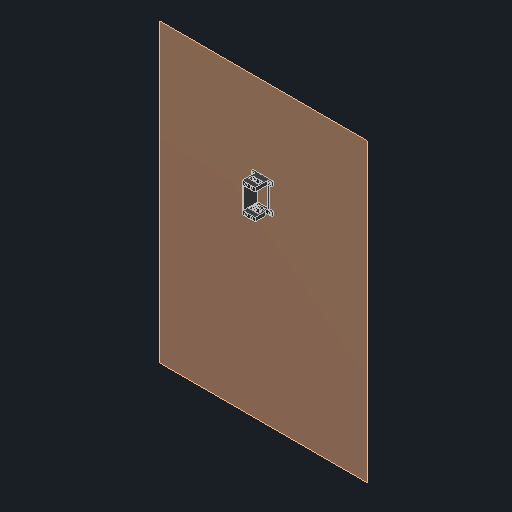
# Autodesk Inventor part: yaw_motor_mount
Saved by Autodesk Inventor 2026.1 (Build 301233020, 233B)
## iProperties
Created: 2025-11-24
Part Number: yaw_motor_mount
Material: 고무, 검은색
Document SubType Name: Modeling
Designer: jaewook
Density: 0.93 g/cm^3
Appearance: 고무 - 검은색
Author: jaewook
Autodesk Inventor part; units mm, degrees
ref_plane "YZ Plane" through (0, 0, 0) normal (1, 0, 0) x (0, 1, 0)
ref_plane "XZ Plane" through (0, 0, 0) normal (0, 1, 0) x (-1, 0, 0)
ref_plane "XY Plane" through (0, 0, 0) normal (0, 0, 1) x (1, 0, 0)
ref_plane "작업 평면1" through (0, 0, -71.9624) normal (0, 0, 1) x (1, 0, 0)
sketch "스케치1" plane through (0, 0, -71.9624) normal (0, 0, 1) x (1, 0, 0)
  line L0 (10, 115.2) -> (10, 75.2) construction
  line L1 (-10, 75.2) -> (-10, 115.2) construction
  line L2 (-10, 115.2) -> (10, 115.2) construction
  line L3 (10, 122.7) -> (-10, 122.7) construction
  line L4 (10, 115.2) -> (10, 122.7) construction
  line L5 (-10, 122.7) -> (-10, 115.2) construction
  circle A0 centre (-4.9, 119.5) radius 2.5 construction
  circle A1 centre (5, 119.5) radius 2.5 construction
  circle A2 centre (5, 70.9) radius 2.5 construction
  circle A3 centre (-4.9, 70.9) radius 2.5 construction
  line L6 (10, 75.2) -> (10, 67.7) construction
  line L7 (10, 67.7) -> (-10, 67.7) construction
  line L8 (-10, 67.7) -> (-10, 75.2) construction
  line L9 (10, 115.2) -> (10, 75.2) projected
  line L10 (-10, 75.2) -> (-10, 115.2) projected
  line L11 (-10, 122.7) -> (-10, 115.2) projected
  line L12 (-10, 115.2) -> (10, 115.2) projected
  line L13 (10, 115.2) -> (10, 122.7) projected
  line L14 (10, 122.7) -> (-10, 122.7) projected
  line L15 (-10, 67.7) -> (-10, 75.2) projected
  line L16 (10, 67.7) -> (-10, 67.7) projected
  line L17 (10, 75.2) -> (10, 67.7) projected
  circle A4 centre (-4.9, 70.9) radius 2.5 projected
  circle A5 centre (5, 70.9) radius 2.5 projected
  line L18 (10, 75.2) -> (-10, 75.2) projected
  circle A6 centre (5, 119.5) radius 2.5 projected
  circle A7 centre (-4.9, 119.5) radius 2.5 projected
  point P0 (0, 0)
ref_plane "작업 평면2" through (0, 0, -71.9624) normal (0, 0, 1) x (1, 0, 0)
sketch "스케치2" plane through (0, 0, -71.9624) normal (0, 0, 1) x (1, 0, 0)
  circle A0 centre (0, 170) radius 2 projected
  circle A1 centre (-73.6122, 42.5) radius 2 projected
  circle A2 centre (73.6122, 42.5) radius 2 projected
  line L0 (-175, 220) -> (-175, 200) projected
  line L1 (-175, 200) -> (-130, 200) projected
  line L2 (-130, 200) -> (-130, 105) projected
  line L3 (-130, 105) -> (-175, 105) projected
  line L4 (-175, 105) -> (-175, -105) projected
  line L5 (-175, -105) -> (-130, -105) projected
  line L6 (-130, -105) -> (-130, -200) projected
  line L7 (-130, -200) -> (-175, -200) projected
  line L8 (-175, -200) -> (-175, -220) projected
  arc A3 (-175, -220) -> (-145, -250) centre (-145, -220) ccw projected
  line L9 (-145, -250) -> (145, -250) projected
  arc A4 (145, -250) -> (175, -220) centre (145, -220) ccw projected
  line L10 (175, -220) -> (175, -200) projected
  line L11 (175, -200) -> (130, -200) projected
  line L12 (130, -200) -> (130, -105) projected
  line L13 (130, -105) -> (175, -105) projected
  line L14 (175, -105) -> (175, 105) projected
  line L15 (175, 105) -> (130, 105) projected
  line L16 (130, 105) -> (130, 200) projected
  line L17 (130, 200) -> (175, 200) projected
  line L18 (175, 200) -> (175, 220) projected
  arc A5 (175, 220) -> (145, 250) centre (145, 220) ccw projected
  line L19 (145, 250) -> (-145, 250) projected
  arc A6 (-145, 250) -> (-175, 220) centre (-145, 220) ccw projected
  circle A7 centre (0, 170) radius 2 projected
  circle A8 centre (-73.6122, 42.5) radius 2 projected
  circle A9 centre (73.6122, 42.5) radius 2 projected
  line L20 (-175, 220) -> (-175, 200) projected
  line L21 (-175, 200) -> (-130, 200) projected
  line L22 (-130, 200) -> (-130, 105) projected
  line L23 (-130, 105) -> (-175, 105) projected
  line L24 (-175, 105) -> (-175, -105) projected
  line L25 (-175, -105) -> (-130, -105) projected
  line L26 (-130, -105) -> (-130, -200) projected
  line L27 (-130, -200) -> (-175, -200) projected
  line L28 (-175, -200) -> (-175, -220) projected
  arc A10 (-175, -220) -> (-145, -250) centre (-145, -220) ccw projected
  line L29 (-145, -250) -> (145, -250) projected
  arc A11 (145, -250) -> (175, -220) centre (145, -220) ccw projected
  line L30 (175, -220) -> (175, -200) projected
  line L31 (175, -200) -> (130, -200) projected
  line L32 (130, -200) -> (130, -105) projected
  line L33 (130, -105) -> (175, -105) projected
  line L34 (175, -105) -> (175, 105) projected
  line L35 (175, 105) -> (130, 105) projected
  line L36 (130, 105) -> (130, 200) projected
  line L37 (130, 200) -> (175, 200) projected
  line L38 (175, 200) -> (175, 220) projected
  arc A12 (175, 220) -> (145, 250) centre (145, 220) ccw projected
  line L39 (145, 250) -> (-145, 250) projected
  arc A13 (-145, 250) -> (-175, 220) centre (-145, 220) ccw projected
  circle A14 centre (0, 170) radius 2 projected
  circle A15 centre (-73.6122, 42.5) radius 2 projected
  circle A16 centre (73.6122, 42.5) radius 2 projected
  line L40 (-175, 220) -> (-175, 200) projected
  line L41 (-175, 200) -> (-130, 200) projected
  line L42 (-130, 200) -> (-130, 105) projected
  line L43 (-130, 105) -> (-175, 105) projected
  line L44 (-175, 105) -> (-175, -105) projected
  line L45 (-175, -105) -> (-130, -105) projected
  line L46 (-130, -105) -> (-130, -200) projected
  line L47 (-130, -200) -> (-175, -200) projected
  line L48 (-175, -200) -> (-175, -220) projected
  arc A17 (-175, -220) -> (-145, -250) centre (-145, -220) ccw projected
  line L49 (-145, -250) -> (145, -250) projected
  arc A18 (145, -250) -> (175, -220) centre (145, -220) ccw projected
  line L50 (175, -220) -> (175, -200) projected
  line L51 (175, -200) -> (130, -200) projected
  line L52 (130, -200) -> (130, -105) projected
  line L53 (130, -105) -> (175, -105) projected
  line L54 (175, -105) -> (175, 105) projected
  line L55 (175, 105) -> (130, 105) projected
  line L56 (130, 105) -> (130, 200) projected
  line L57 (130, 200) -> (175, 200) projected
  line L58 (175, 200) -> (175, 220) projected
  arc A19 (175, 220) -> (145, 250) centre (145, 220) ccw projected
  line L59 (145, 250) -> (-145, 250) projected
  arc A20 (-145, 250) -> (-175, 220) centre (-145, 220) ccw projected
  circle A21 centre (-4.9, 70.9) radius 2.5 projected
  circle A22 centre (-4.9, 70.9) radius 2.5 projected
  circle A23 centre (5, 70.9) radius 2.5 projected
  circle A24 centre (5, 119.5) radius 2.5 projected
  circle A25 centre (-4.9, 119.5) radius 2.5 projected
  arc A26 (175, 220) -> (145, 250) centre (145, 220) ccw projected
  line L60 (-145, 250) -> (145, 250) projected
  arc A27 (-145, 250) -> (-175, 220) centre (-145, 220) ccw projected
  line L61 (-175, -220) -> (-175, 220) projected
  arc A28 (-175, -220) -> (-145, -250) centre (-145, -220) ccw projected
  line L62 (145, -250) -> (-145, -250) projected
  arc A29 (145, -250) -> (175, -220) centre (145, -220) ccw projected
  line L63 (175, 220) -> (175, -220) projected
  circle A30 centre (0, -175) radius 36 projected
  circle A31 centre (0, 85) radius 103.75 projected
  line L64 (10, 75.2) -> (-10, 75.2)
  line L65 (-10, 75.2) -> (-10, 115.2)
  line L66 (-10, 115.2) -> (10, 115.2)
  line L67 (10, 115.2) -> (10, 75.2)
  line L68 (10.3, 74.9) -> (10.3, 115.5)
  line L69 (10.3, 115.5) -> (-10.3, 115.5)
  line L70 (-10.3, 115.5) -> (-10.3, 74.9)
  line L71 (-10.3, 74.9) -> (10.3, 74.9)
  line L72 (12, 67.7) -> (-12, 67.7)
  line L73 (-12, 67.7) -> (-12, 122.7)
  line L74 (-12, 122.7) -> (12, 122.7)
  line L75 (12, 122.7) -> (12, 67.7)
  line L76 (10, 95.2) -> (-10, 95.2) construction
  line L77 (0, 95.2) -> (0, 75.2) construction
  line L78 (10.3, 74.9) -> (12, 74.9)
  line L79 (10.3, 115.5) -> (12, 115.5)
  circle A32 centre (-4.9, 119.5) radius 2
  circle A33 centre (5, 119.5) radius 2
  circle A34 centre (-4.9, 70.9) radius 2
  circle A35 centre (5, 70.9) radius 2
  circle A36 centre (-123, 166.7672) radius 2 projected
  circle A37 centre (122.9975, 135.7594) radius 2 projected
  circle A38 centre (97.9975, -135.761) radius 2 projected
  circle A39 centre (15.5, 71.3) radius 2 projected
  circle A40 centre (165.0067, -210) radius 2.5 projected
  circle A41 centre (119.0003, -180.2596) radius 1.25 projected
  circle A42 centre (-119, -122.2672) radius 1.25 projected
  circle A43 centre (-123, -135.7672) radius 2 projected
  circle A44 centre (0.0196, 140) radius 2 projected
  circle A45 centre (-123, -166.7672) radius 2 projected
  circle A46 centre (-70, -122.2672) radius 1.25 projected
  circle A47 centre (69.9966, -122.2627) radius 1.25 projected
  circle A48 centre (-165, 0) radius 2.5 projected
  circle A49 centre (-165.0067, 210) radius 2.5 projected
  circle A50 centre (-15.5, 119.1) radius 2 projected
  circle A51 centre (97.9995, -166.761) radius 2 projected
  circle A52 centre (97.9995, 166.761) radius 2 projected
  circle A53 centre (-98, 166.7672) radius 2 projected
  circle A54 centre (-123, 135.7672) radius 2 projected
  circle A55 centre (97.9975, 135.761) radius 2 projected
  circle A56 centre (122.9975, -135.7594) radius 2 projected
  circle A57 centre (-15.5, 71.3) radius 2 projected
  circle A58 centre (-164.9933, -210) radius 2.5 projected
  circle A59 centre (70.0003, -180.2627) radius 1.25 projected
  circle A60 centre (-119, -180.2672) radius 1.25 projected
  circle A61 centre (-98, -135.7672) radius 2 projected
  circle A62 centre (47.6216, 57.483) radius 2 projected
  circle A63 centre (-47.6412, 57.517) radius 2 projected
  circle A64 centre (-98, -166.7672) radius 2 projected
  circle A65 centre (-70, -180.2672) radius 1.25 projected
  circle A66 centre (118.9966, -122.2596) radius 1.25 projected
  circle A67 centre (165, 0) radius 2.5 projected
  circle A68 centre (164.9933, 210) radius 2.5 projected
  circle A69 centre (15.5, 119.1) radius 2 projected
  circle A70 centre (122.9995, -166.7594) radius 2 projected
  circle A71 centre (122.9995, 166.7594) radius 2 projected
  circle A72 centre (-98, 135.7672) radius 2 projected
  circle A73 centre (-123, 166.7672) radius 2 projected
  circle A74 centre (122.9975, 135.7594) radius 2 projected
  circle A75 centre (97.9975, -135.761) radius 2 projected
  circle A76 centre (15.5, 71.3) radius 2 projected
  circle A77 centre (165.0067, -210) radius 2.5 projected
  circle A78 centre (119.0003, -180.2596) radius 1.25 projected
  circle A79 centre (-119, -122.2672) radius 1.25 projected
  circle A80 centre (-123, -135.7672) radius 2 projected
  circle A81 centre (0.0196, 140) radius 2 projected
  circle A82 centre (-123, -166.7672) radius 2 projected
  circle A83 centre (-70, -122.2672) radius 1.25 projected
  circle A84 centre (69.9966, -122.2627) radius 1.25 projected
  circle A85 centre (-165, 0) radius 2.5 projected
  circle A86 centre (-165.0067, 210) radius 2.5 projected
  circle A87 centre (-15.5, 119.1) radius 2 projected
  circle A88 centre (97.9995, -166.761) radius 2 projected
  circle A89 centre (97.9995, 166.761) radius 2 projected
  circle A90 centre (-98, 166.7672) radius 2 projected
  circle A91 centre (-123, 135.7672) radius 2 projected
  circle A92 centre (97.9975, 135.761) radius 2 projected
  circle A93 centre (122.9975, -135.7594) radius 2 projected
  circle A94 centre (-15.5, 71.3) radius 2 projected
  circle A95 centre (-164.9933, -210) radius 2.5 projected
  circle A96 centre (70.0003, -180.2627) radius 1.25 projected
  circle A97 centre (-119, -180.2672) radius 1.25 projected
  circle A98 centre (-98, -135.7672) radius 2 projected
  circle A99 centre (47.6216, 57.483) radius 2 projected
  circle A100 centre (-47.6412, 57.517) radius 2 projected
  circle A101 centre (-98, -166.7672) radius 2 projected
  circle A102 centre (-70, -180.2672) radius 1.25 projected
  circle A103 centre (118.9966, -122.2596) radius 1.25 projected
  circle A104 centre (165, 0) radius 2.5 projected
  circle A105 centre (164.9933, 210) radius 2.5 projected
  circle A106 centre (15.5, 119.1) radius 2 projected
  circle A107 centre (122.9995, -166.7594) radius 2 projected
  circle A108 centre (122.9995, 166.7594) radius 2 projected
  circle A109 centre (-98, 135.7672) radius 2 projected
  circle A110 centre (-123, 166.7672) radius 2 projected
  circle A111 centre (122.9975, 135.7594) radius 2 projected
  circle A112 centre (97.9975, -135.761) radius 2 projected
  circle A113 centre (15.5, 71.3) radius 2 projected
  circle A114 centre (165.0067, -210) radius 2.5 projected
  circle A115 centre (119.0003, -180.2596) radius 1.25 projected
  circle A116 centre (-119, -122.2672) radius 1.25 projected
  circle A117 centre (-123, -135.7672) radius 2 projected
  circle A118 centre (0.0196, 140) radius 2 projected
  circle A119 centre (-123, -166.7672) radius 2 projected
  circle A120 centre (-70, -122.2672) radius 1.25 projected
  circle A121 centre (69.9966, -122.2627) radius 1.25 projected
  circle A122 centre (-165, 0) radius 2.5 projected
  circle A123 centre (-165.0067, 210) radius 2.5 projected
  circle A124 centre (-15.5, 119.1) radius 2 projected
  circle A125 centre (97.9995, -166.761) radius 2 projected
  circle A126 centre (97.9995, 166.761) radius 2 projected
  circle A127 centre (-98, 166.7672) radius 2 projected
  circle A128 centre (-123, 135.7672) radius 2 projected
  circle A129 centre (97.9975, 135.761) radius 2 projected
  circle A130 centre (122.9975, -135.7594) radius 2 projected
  circle A131 centre (-15.5, 71.3) radius 2 projected
  circle A132 centre (-164.9933, -210) radius 2.5 projected
  circle A133 centre (70.0003, -180.2627) radius 1.25 projected
  circle A134 centre (-119, -180.2672) radius 1.25 projected
  circle A135 centre (-98, -135.7672) radius 2 projected
  circle A136 centre (47.6216, 57.483) radius 2 projected
  circle A137 centre (-47.6412, 57.517) radius 2 projected
  circle A138 centre (-98, -166.7672) radius 2 projected
  circle A139 centre (-70, -180.2672) radius 1.25 projected
  circle A140 centre (118.9966, -122.2596) radius 1.25 projected
  circle A141 centre (165, 0) radius 2.5 projected
  circle A142 centre (164.9933, 210) radius 2.5 projected
  circle A143 centre (15.5, 119.1) radius 2 projected
  circle A144 centre (122.9995, -166.7594) radius 2 projected
  circle A145 centre (122.9995, 166.7594) radius 2 projected
  circle A146 centre (-98, 135.7672) radius 2 projected
  line L80 (-110, 97.5) -> (-93, 97.5) projected
  line L81 (-93, 97.5) -> (-93, 89.5) projected
  line L82 (-93, 89.5) -> (-110, 89.5) projected
  line L83 (-110, 89.5) -> (-110, 97.5) projected
  circle A147 centre (148, -23.75) radius 2 projected
  circle A148 centre (130.626, -27.584) radius 1.5 projected
  circle A149 centre (118.5, 61.5) radius 1.5 projected
  circle A150 centre (-118.5, 61.5) radius 1.5 projected
  circle A151 centre (21, -158.9548) radius 2 projected
  circle A152 centre (-22, -53) radius 2 projected
  circle A153 centre (-49.5, -194.9548) radius 2 projected
  circle A154 centre (-49.5, -158.9548) radius 2 projected
  circle A155 centre (21, -194.9548) radius 2 projected
  circle A156 centre (-155, 25) radius 1.5 projected
  circle A157 centre (118.5, 25) radius 1.5 projected
  circle A158 centre (123.133, -76) radius 1.5 projected
  circle A159 centre (37, -84) radius 2 projected
  line L84 (-93, -89.5) -> (-93, -97.5) projected
  line L85 (-93, -97.5) -> (-110, -97.5) projected
  line L86 (-110, -97.5) -> (-110, -89.5) projected
  line L87 (-110, -89.5) -> (-93, -89.5) projected
  circle A160 centre (-130, 5) radius 6 projected
  line L88 (110, 89.5) -> (93, 89.5) projected
  line L89 (93, 89.5) -> (93, 97.5) projected
  line L90 (93, 97.5) -> (110, 97.5) projected
  line L91 (110, 97.5) -> (110, 89.5) projected
  circle A161 centre (148, -84) radius 2 projected
  circle A162 centre (47.999, -27.584) radius 1.5 projected
  circle A163 centre (155, 61.5) radius 1.5 projected
  circle A164 centre (-155, 61.5) radius 1.5 projected
  circle A165 centre (49.5, -158.9548) radius 2 projected
  circle A166 centre (-86, -93.5) radius 2 projected
  circle A167 centre (-21, -194.9548) radius 2 projected
  circle A168 centre (-150, -53) radius 2 projected
  circle A169 centre (-21, -158.9548) radius 2 projected
  circle A170 centre (49.5, -194.9548) radius 2 projected
  circle A171 centre (-118.5, 25) radius 1.5 projected
  circle A172 centre (155, 25) radius 1.5 projected
  circle A173 centre (48, -76) radius 1.5 projected
  circle A174 centre (37, -23.75) radius 2 projected
  line L92 (110, -89.5) -> (110, -97.5) projected
  line L93 (110, -97.5) -> (93, -97.5) projected
  line L94 (93, -97.5) -> (93, -89.5) projected
  line L95 (93, -89.5) -> (110, -89.5) projected
  circle A175 centre (-70, 5) radius 6 projected
  line L96 (-110, 97.5) -> (-93, 97.5) projected
  line L97 (-93, 97.5) -> (-93, 89.5) projected
  line L98 (-93, 89.5) -> (-110, 89.5) projected
  line L99 (-110, 89.5) -> (-110, 97.5) projected
  circle A176 centre (148, -23.75) radius 2 projected
  circle A177 centre (130.626, -27.584) radius 1.5 projected
  circle A178 centre (118.5, 61.5) radius 1.5 projected
  circle A179 centre (-118.5, 61.5) radius 1.5 projected
  circle A180 centre (21, -158.9548) radius 2 projected
  circle A181 centre (-22, -53) radius 2 projected
  circle A182 centre (-49.5, -194.9548) radius 2 projected
  circle A183 centre (-49.5, -158.9548) radius 2 projected
  circle A184 centre (21, -194.9548) radius 2 projected
  circle A185 centre (-155, 25) radius 1.5 projected
  circle A186 centre (118.5, 25) radius 1.5 projected
  circle A187 centre (123.133, -76) radius 1.5 projected
  circle A188 centre (37, -84) radius 2 projected
  line L100 (-93, -89.5) -> (-93, -97.5) projected
  line L101 (-93, -97.5) -> (-110, -97.5) projected
  line L102 (-110, -97.5) -> (-110, -89.5) projected
  line L103 (-110, -89.5) -> (-93, -89.5) projected
  circle A189 centre (-130, 5) radius 6 projected
  line L104 (110, 89.5) -> (93, 89.5) projected
  line L105 (93, 89.5) -> (93, 97.5) projected
  line L106 (93, 97.5) -> (110, 97.5) projected
  line L107 (110, 97.5) -> (110, 89.5) projected
  circle A190 centre (148, -84) radius 2 projected
  circle A191 centre (47.999, -27.584) radius 1.5 projected
  circle A192 centre (155, 61.5) radius 1.5 projected
  circle A193 centre (-155, 61.5) radius 1.5 projected
  circle A194 centre (49.5, -158.9548) radius 2 projected
  circle A195 centre (-86, -93.5) radius 2 projected
  circle A196 centre (-21, -194.9548) radius 2 projected
  circle A197 centre (-150, -53) radius 2 projected
  circle A198 centre (-21, -158.9548) radius 2 projected
  circle A199 centre (49.5, -194.9548) radius 2 projected
  circle A200 centre (-118.5, 25) radius 1.5 projected
  circle A201 centre (155, 25) radius 1.5 projected
  circle A202 centre (48, -76) radius 1.5 projected
  circle A203 centre (37, -23.75) radius 2 projected
  line L108 (110, -89.5) -> (110, -97.5) projected
  line L109 (110, -97.5) -> (93, -97.5) projected
  line L110 (93, -97.5) -> (93, -89.5) projected
  line L111 (93, -89.5) -> (110, -89.5) projected
  circle A204 centre (-70, 5) radius 6 projected
  line L112 (-110, 97.5) -> (-93, 97.5) projected
  line L113 (-93, 97.5) -> (-93, 89.5) projected
  line L114 (-93, 89.5) -> (-110, 89.5) projected
  line L115 (-110, 89.5) -> (-110, 97.5) projected
  circle A205 centre (148, -23.75) radius 2 projected
  circle A206 centre (130.626, -27.584) radius 1.5 projected
  circle A207 centre (118.5, 61.5) radius 1.5 projected
  circle A208 centre (-118.5, 61.5) radius 1.5 projected
  circle A209 centre (21, -158.9548) radius 2 projected
  circle A210 centre (-22, -53) radius 2 projected
  circle A211 centre (-49.5, -194.9548) radius 2 projected
  circle A212 centre (-49.5, -158.9548) radius 2 projected
  circle A213 centre (21, -194.9548) radius 2 projected
  circle A214 centre (-155, 25) radius 1.5 projected
  circle A215 centre (118.5, 25) radius 1.5 projected
  circle A216 centre (123.133, -76) radius 1.5 projected
  circle A217 centre (37, -84) radius 2 projected
  line L116 (-93, -89.5) -> (-93, -97.5) projected
  line L117 (-93, -97.5) -> (-110, -97.5) projected
  line L118 (-110, -97.5) -> (-110, -89.5) projected
  line L119 (-110, -89.5) -> (-93, -89.5) projected
  circle A218 centre (-130, 5) radius 6 projected
  line L120 (110, 89.5) -> (93, 89.5) projected
  line L121 (93, 89.5) -> (93, 97.5) projected
  line L122 (93, 97.5) -> (110, 97.5) projected
  line L123 (110, 97.5) -> (110, 89.5) projected
  circle A219 centre (148, -84) radius 2 projected
  circle A220 centre (47.999, -27.584) radius 1.5 projected
  circle A221 centre (155, 61.5) radius 1.5 projected
  circle A222 centre (-155, 61.5) radius 1.5 projected
  circle A223 centre (49.5, -158.9548) radius 2 projected
  circle A224 centre (-86, -93.5) radius 2 projected
  circle A225 centre (-21, -194.9548) radius 2 projected
  circle A226 centre (-150, -53) radius 2 projected
  circle A227 centre (-21, -158.9548) radius 2 projected
  circle A228 centre (49.5, -194.9548) radius 2 projected
  circle A229 centre (-118.5, 25) radius 1.5 projected
  circle A230 centre (155, 25) radius 1.5 projected
  circle A231 centre (48, -76) radius 1.5 projected
  circle A232 centre (37, -23.75) radius 2 projected
  line L124 (110, -89.5) -> (110, -97.5) projected
  line L125 (110, -97.5) -> (93, -97.5) projected
  line L126 (93, -97.5) -> (93, -89.5) projected
  line L127 (93, -89.5) -> (110, -89.5) projected
  circle A233 centre (-70, 5) radius 6 projected
  circle A234 centre (0, -216.4634) radius 1.5 projected
  circle A235 centre (28.4775, -136.4634) radius 1.5 projected
  circle A236 centre (-28.4775, -136.4634) radius 1.5 projected
  circle A237 centre (0, -216.4634) radius 1.5 projected
  circle A238 centre (28.4775, -136.4634) radius 1.5 projected
  circle A239 centre (-28.4775, -136.4634) radius 1.5 projected
  circle A240 centre (0, -216.4634) radius 1.5 projected
  circle A241 centre (28.4775, -136.4634) radius 1.5 projected
  circle A242 centre (-28.4775, -136.4634) radius 1.5 projected
  circle A243 centre (-165, 210) radius 2.5 projected
  circle A244 centre (165, 210) radius 2.5 projected
  circle A245 centre (-165, 0) radius 2.5 projected
  circle A246 centre (165, 0) radius 2.5 projected
  circle A247 centre (165, -210) radius 2.5 projected
  circle A248 centre (-165, -210) radius 2.5 projected
  point P0 (0, 0)
  point P1 (10, 67.7)
  dimension "d4" = 0.3
  dimension "d5" = 0.3
  dimension "d6" = 0.3
  dimension "d7" = 55
  dimension "d8" = 2
  dimension "d9" = 27.5
  dimension "d23" = 4
  dimension "d24" = 4
  dimension "d25" = 4
  dimension "d26" = 4
  constraints: 32 end point, 11 perpendicular, 4 centre point, 4 coincident, 4 midpoint, 3 point on line, 2 horizontal, 2 parallel, 2 other
  measures "d4" distance between parallel lines of L65 L70
  measures "d5" distance between parallel lines of L64 L71
  measures "d6" distance between parallel lines of L67 L68
  measures "d7" distance of L72.end L73.end
  measures "d8" distance between parallel lines of L75 L67
  measures "d9" distance from line of L77.start L72
  measures "d23" diameter of A32
  measures "d24" diameter of A33
  measures "d25" diameter of A34
  measures "d26" diameter of A35
extrude "돌출1" add sketch "스케치2" along normal blind 27.3 contours A21 | A23 | A24 | A25 | L78 L75 L72 L73 L74 L79 L69 L70 L71 | A32 | A33 | A34 | A35
sketch "스케치3" plane through (12, 67.7, -71.9624) normal (1, 0, 0) x (0, 0, -1)
  line L0 (0, 0) -> (0, 7.2) projected
  line L1 (0, 7.2) -> (-27.3, 7.2) projected
  line L2 (0, 0) -> (-27.3, 0) projected
  line L3 (-8.5, 0) -> (-3.5, 0)
  line L4 (-3.5, 0) -> (-3.5, 7.2)
  line L5 (-3.5, 7.2) -> (-8.5, 7.2)
  line L6 (-8.5, 7.2) -> (-8.5, 0)
  point P0 (-71.9624, -67.7)
  point P1 (-8.5, 0)
  point P2 (-3.5, 0)
  dimension "d12" = 5
  dimension "d13" = 3.5
  constraints: 8 end point, 2 parallel, 1 horizontal, 1 perpendicular, 1 point on line
  measures "d12" distance between parallel lines of L4 L6
  measures "d13" distance between parallel lines of L0 L4
extrude "돌출2" cut sketch "스케치3" against normal blind 21 contours L2 L6 L1 L4
sketch "스케치4" plane through (0, 0, -71.9624) normal (0, 0, -1) x (-1, 0, 0)
  line L0 (-12, 74.9) -> (10.3, 74.9) projected
  line L1 (-12, 67.7) -> (-12, 74.9) projected
  line L2 (12, 67.7) -> (-12, 67.7) projected
  line L3 (12, 122.7) -> (12, 67.7) projected
  line L4 (-12, 115.5) -> (-12, 122.7) projected
  line L5 (-12, 67.7) -> (-19, 67.7)
  line L6 (-19, 67.7) -> (-19, 74.9)
  line L7 (-19, 74.9) -> (-12, 74.9)
  line L8 (-12, 74.9) -> (-12, 67.7)
  circle A0 centre (-15.5, 71.3) radius 2
  line L9 (0, 67.7) -> (0, 122.7) construction
  line L10 (-12, 122.7) -> (12, 122.7) projected
  line L11 (-10, 95.2) -> (12, 95.2) construction
  line L12 (-10, 115.2) -> (-10, 75.2) construction
  line L13 (-12, 122.7) -> (-12, 115.5)
  line L14 (-12, 122.7) -> (-19, 122.7)
  line L15 (-19, 122.7) -> (-19, 115.5)
  line L16 (-19, 115.5) -> (-12, 115.5)
  circle A1 centre (-15.5, 119.1) radius 2
  line L17 (12, 67.7) -> (12, 74.9)
  line L18 (12, 115.5) -> (12, 122.7)
  line L19 (12, 67.7) -> (19, 67.7)
  line L20 (19, 67.7) -> (19, 74.9)
  line L21 (19, 74.9) -> (12, 74.9)
  line L22 (12, 74.9) -> (12, 67.7)
  circle A2 centre (15.5, 71.3) radius 2
  line L23 (19, 115.5) -> (12, 115.5)
  line L24 (19, 122.7) -> (19, 115.5)
  line L25 (12, 122.7) -> (19, 122.7)
  circle A3 centre (15.5, 119.1) radius 2
  line L26 (12, 122.7) -> (12, 115.5)
  point P0 (0, 0)
  point P1 (-12, 115.5)
  point P2 (-12, 74.9)
  dimension "d16" = 7
  dimension "d18" = 4
  dimension "d19" = 3.6
  dimension "d20" = 3.5
  constraints: 40 end point, 16 symmetric about line, 4 centre point, 4 midpoint, 2 parallel, 2 perpendicular, 1 collinear, 1 horizontal, 3 other
  measures "d16" distance of L6.end L7.end
  measures "d18" diameter of A0
  measures "d19" distance from line of A0.centre L7
  measures "d20" distance from line of A0.centre L6
extrude "돌출3" add sketch "스케치4" against normal blind 3.5
ref_plane "작업 평면3" through (0, 0, -71.9624) normal (0, 0, 1) x (1, 0, 0)
extrude "돌출4" cut sketch "스케치1" along normal through all contours A4 | A5 | A6 | A7
sketch "스케치5" plane through (-12, 67.7, -44.6624) normal (0, -1, 0) x (1, 0, 0)
  line L0 (3, -18.8) -> (24, -18.8) projected
  line L1 (24, -18.8) -> (24, 0) projected
  line L2 (3, -18.8) -> (24, -18.8)
  line L3 (24, -18.8) -> (24, -8.8)
  line L4 (24, -8.8) -> (3, -8.8)
  line L5 (3, -8.8) -> (3, -16.8)
  line L6 (3, -23.8) -> (3, -18.8) projected
  line L7 (3, -16.8) -> (24, -16.8)
  point P0 (12, 44.6624)
  dimension "d36" = 2
  dimension "d37" = 8
  constraints: 10 end point, 2 parallel, 2 perpendicular, 2 point on line, 1 collinear, 1 horizontal
  measures "d36" distance between parallel lines of L0 L7
  measures "d37" distance of L4.end L5.end
extrude "돌출5" cut sketch "스케치5" against normal through all
sketch "스케치6" plane through (0, 0, -71.9624) normal (0, 0, -1) x (-1, 0, 0)
  line L0 (10.3, 115.5) -> (-19, 115.5) projected
  line L1 (10.3, 74.9) -> (-19, 74.9) projected
  line L2 (-19, 67.7) -> (19, 67.7) projected
  line L3 (-12, 122.7) -> (12, 122.7) projected
  line L4 (0, 122.7) -> (0, 67.7) construction
  line L5 (-10.3, 74.9) -> (-10.3, 115.5)
  line L6 (-12, 115.5) -> (-12, 74.9)
  point P0 (12, 74.9)
  point P1 (12, 115.5)
  point P2 (0, 0)
  point P3 (-10.3, 115.5)
  point P4 (-12, 74.9)
  constraints: 6 end point, 4 symmetric about line, 2 midpoint
extrude "돌출6" add sketch "스케치6" against normal blind 3.5
sketch "스케치7" plane through (-12, 122.7, -44.6624) normal (0, 1, 0) x (1, 0, 0)
  line L0 (24, 8.8) -> (3, 8.8) projected
  line L1 (3, 8.8) -> (3, 16.8) projected
  line L2 (3, 18.8) -> (24, 18.8) projected
  line L3 (0, 23.8) -> (0, 0) projected
  line L4 (24, 0) -> (0, 0) projected
  line L5 (12, -44.6624) -> (12, 0) construction
  line L6 (21, 8.8) -> (21, 18.8)
  line L7 (24, 23.8) -> (24, 0)
  point P0 (24, 8.8)
  constraints: 6 end point, 2 symmetric about line, 1 midpoint
extrude "돌출7" add sketch "스케치7" against normal up to surface (7.2 mm away)
sketch "스케치8" plane through (-12, 67.7, -44.6624) normal (0, -1, 0) x (1, 0, 0)
  line L0 (24, -16.8) -> (3, -16.8) projected
  line L1 (3, -8.8) -> (24, -8.8) projected
  line L2 (21, -16.8) -> (21, -8.8) projected
  line L3 (24, -23.8) -> (24, 0) projected
  line L4 (24, -23.8) -> (24, -27.3) projected
  point P0 (12, 44.6624)
extrude "돌출8" add sketch "스케치8" against normal up to surface (7.2 mm away)
